Autodesk Inventor part; units mm, degrees
(part 6 of 6)
  line L4439 (-10.0121, 28.4168) -> (-10.0047, 28.6447)
  line L4440 (-10.0047, 28.6447) -> (-9.9918, 28.8863)
  line L4441 (-9.9918, 28.8863) -> (-9.973, 29.1388)
  line L4442 (-9.973, 29.1388) -> (-9.9523, 29.359)
  arc A136 (-9.2052, 29.6018) -> (-9.9523, 29.359) centre (0, 0) ccw
  line L4443 (-9.2052, 29.6018) -> (-9.059, 29.4358)
  line L4444 (-9.059, 29.4358) -> (-8.8954, 29.2425)
  line L4445 (-8.8954, 29.2425) -> (-8.7429, 29.0547)
  line L4446 (-8.7429, 29.0547) -> (-8.603, 28.8746)
  line L4447 (-8.603, 28.8746) -> (-8.4737, 28.7009)
  line L4448 (-8.4737, 28.7009) -> (-8.3547, 28.5338)
  line L4449 (-8.3547, 28.5338) -> (-8.2472, 28.3759)
  line L4450 (-8.2472, 28.3759) -> (-8.1494, 28.2257)
  line L4451 (-8.1494, 28.2257) -> (-7.9652, 27.9266)
  line L4452 (-7.9652, 27.9266) -> (-7.9351, 27.8907)
  line L4453 (-7.9351, 27.8907) -> (-7.9073, 27.8683)
  line L4454 (-7.9073, 27.8683) -> (-7.8823, 27.8592)
  line L4455 (-7.8823, 27.8592) -> (-7.8657, 27.861)
  line L4456 (-7.8657, 27.861) -> (-7.4928, 27.9636)
  line L4457 (-7.4928, 27.9636) -> (-7.1186, 28.0612)
  line L4458 (-7.1186, 28.0612) -> (-7.1033, 28.0679)
  line L4459 (-7.1033, 28.0679) -> (-7.0862, 28.0883)
  line L4460 (-7.0862, 28.0883) -> (-7.0733, 28.1216)
  line L4461 (-7.0733, 28.1216) -> (-7.0652, 28.1677)
  line L4462 (-7.0652, 28.1677) -> (-7.0553, 28.5189)
  line L4463 (-7.0553, 28.5189) -> (-7.0457, 28.6979)
  line L4464 (-7.0457, 28.6979) -> (-7.0315, 28.8883)
  line L4465 (-7.0315, 28.8883) -> (-7.012, 29.0926)
  line L4466 (-7.012, 29.0926) -> (-6.9869, 29.3077)
  line L4467 (-6.9869, 29.3077) -> (-6.9557, 29.5336)
  line L4468 (-6.9557, 29.5336) -> (-6.9177, 29.7725)
  line L4469 (-6.9177, 29.7725) -> (-6.8726, 30.0216)
  line L4470 (-6.8726, 30.0216) -> (-6.829, 30.2385)
  arc A137 (-6.0605, 30.4018) -> (-6.829, 30.2385) centre (0, 0) ccw
  line L4471 (-6.0605, 30.4018) -> (-5.9325, 30.2214)
  line L4472 (-5.9325, 30.2214) -> (-5.79, 30.0122)
  line L4473 (-5.79, 30.0122) -> (-5.658, 29.8094)
  line L4474 (-5.658, 29.8094) -> (-5.5376, 29.6157)
  line L4475 (-5.5376, 29.6157) -> (-5.4272, 29.4294)
  line L4476 (-5.4272, 29.4294) -> (-5.3263, 29.2508)
  line L4477 (-5.3263, 29.2508) -> (-5.2359, 29.0826)
  line L4478 (-5.2359, 29.0826) -> (-5.1544, 28.9229)
  line L4479 (-5.1544, 28.9229) -> (-5.0025, 28.6062)
  line L4480 (-5.0025, 28.6062) -> (-4.9763, 28.5674)
  line L4481 (-4.9763, 28.5674) -> (-4.951, 28.5421)
  line L4482 (-4.951, 28.5421) -> (-4.927, 28.5305)
  line L4483 (-4.927, 28.5305) -> (-4.9104, 28.5306)
  line L4484 (-4.9104, 28.5306) -> (-4.5288, 28.5936)
  line L4485 (-4.5288, 28.5936) -> (-4.1464, 28.6516)
  line L4486 (-4.1464, 28.6516) -> (-4.1305, 28.6567)
  line L4487 (-4.1305, 28.6567) -> (-4.1114, 28.6751)
  line L4488 (-4.1114, 28.6751) -> (-4.0951, 28.7069)
  line L4489 (-4.0951, 28.7069) -> (-4.0822, 28.7519)
  line L4490 (-4.0822, 28.7519) -> (-4.0356, 29.1001)
  line L4491 (-4.0356, 29.1001) -> (-4.0074, 29.2771)
  line L4492 (-4.0074, 29.2771) -> (-3.9734, 29.465)
  line L4493 (-3.9734, 29.465) -> (-3.9326, 29.6661)
  line L4494 (-3.9326, 29.6661) -> (-3.8852, 29.8774)
  line L4495 (-3.8852, 29.8774) -> (-3.8305, 30.0989)
  line L4496 (-3.8305, 30.0989) -> (-3.7677, 30.3325)
  line L4497 (-3.7677, 30.3325) -> (-3.6968, 30.5755)
  line L4498 (-3.6968, 30.5755) -> (-3.6308, 30.7866)
  arc A138 (-2.8495, 30.8688) -> (-3.6308, 30.7866) centre (0, 0) ccw
  line L4499 (-2.8495, 30.8688) -> (-2.741, 30.676)
  line L4500 (-2.741, 30.676) -> (-2.6211, 30.453)
  line L4501 (-2.6211, 30.453) -> (-2.5111, 30.2376)
  line L4502 (-2.5111, 30.2376) -> (-2.4116, 30.0323)
  line L4503 (-2.4116, 30.0323) -> (-2.3213, 29.8355)
  line L4504 (-2.3213, 29.8355) -> (-2.2396, 29.6473)
  line L4505 (-2.2396, 29.6473) -> (-2.1673, 29.4705)
  line L4506 (-2.1673, 29.4705) -> (-2.1029, 29.3033)
  line L4507 (-2.1029, 29.3033) -> (-1.9849, 28.9724)
  line L4508 (-1.9849, 28.9724) -> (-1.9629, 28.931)
  line L4509 (-1.9629, 28.931) -> (-1.9404, 28.9033)
  line L4510 (-1.9404, 28.9033) -> (-1.9178, 28.8892)
  line L4511 (-1.9178, 28.8892) -> (-1.9012, 28.8876)
  line L4512 (-1.9012, 28.8876) -> (-1.5151, 28.9103)
  line L4513 (-1.5151, 28.9103) -> (-1.1288, 28.9281)
  line L4514 (-1.1288, 28.9281) -> (-1.1124, 28.9314)
  line L4515 (-1.1124, 28.9314) -> (-1.0915, 28.9478)
  line L4516 (-1.0915, 28.9478) -> (-1.0719, 28.9777)
  line L4517 (-1.0719, 28.9777) -> (-1.0544, 29.0211)
  line L4518 (-1.0544, 29.0211) -> (-0.9717, 29.3626)
  line L4519 (-0.9717, 29.3626) -> (-0.9251, 29.5356)
  line L4520 (-0.9251, 29.5356) -> (-0.8717, 29.719)
  line L4521 (-0.8717, 29.719) -> (-0.8101, 29.9147)
  line L4522 (-0.8101, 29.9147) -> (-0.7408, 30.1199)
  line L4523 (-0.7408, 30.1199) -> (-0.6634, 30.3344)
  line L4524 (-0.6634, 30.3344) -> (-0.5765, 30.5601)
  line L4525 (-0.5765, 30.5601) -> (-0.4805, 30.7945)
  line L4526 (-0.4805, 30.7945) -> (-0.3928, 30.9975)
  arc A139 (0.3928, 30.9975) -> (-0.3928, 30.9975) centre (0, 0) ccw
  line L4527 (0.3928, 30.9975) -> (0.4805, 30.7945)
  line L4528 (0.4805, 30.7945) -> (0.5765, 30.5601)
  line L4529 (0.5765, 30.5601) -> (0.6634, 30.3344)
  line L4530 (0.6634, 30.3344) -> (0.7408, 30.1199)
  line L4531 (0.7408, 30.1199) -> (0.8101, 29.9147)
  line L4532 (0.8101, 29.9147) -> (0.8717, 29.719)
  line L4533 (0.8717, 29.719) -> (0.9251, 29.5356)
  line L4534 (0.9251, 29.5356) -> (0.9717, 29.3626)
  line L4535 (0.9717, 29.3626) -> (1.0544, 29.0211)
  line L4536 (1.0544, 29.0211) -> (1.0719, 28.9777)
  line L4537 (1.0719, 28.9777) -> (1.0915, 28.9478)
  line L4538 (1.0915, 28.9478) -> (1.1124, 28.9314)
  line L4539 (1.1124, 28.9314) -> (1.1288, 28.9281)
  line L4540 (1.1288, 28.9281) -> (1.5151, 28.9103)
  line L4541 (1.5151, 28.9103) -> (1.9012, 28.8876)
  line L4542 (1.9012, 28.8876) -> (1.9178, 28.8892)
  line L4543 (1.9178, 28.8892) -> (1.9404, 28.9033)
  line L4544 (1.9404, 28.9033) -> (1.9629, 28.931)
  line L4545 (1.9629, 28.931) -> (1.9849, 28.9724)
  line L4546 (1.9849, 28.9724) -> (2.1029, 29.3033)
  line L4547 (2.1029, 29.3033) -> (2.1673, 29.4705)
  line L4548 (2.1673, 29.4705) -> (2.2396, 29.6473)
  line L4549 (2.2396, 29.6473) -> (2.3213, 29.8355)
  line L4550 (2.3213, 29.8355) -> (2.4116, 30.0323)
  line L4551 (2.4116, 30.0323) -> (2.5111, 30.2376)
  line L4552 (2.5111, 30.2376) -> (2.6211, 30.453)
  line L4553 (2.6211, 30.453) -> (2.741, 30.676)
  line L4554 (2.741, 30.676) -> (2.8495, 30.8688)
  arc A140 (3.6308, 30.7866) -> (2.8495, 30.8688) centre (0, 0) ccw
  line L4555 (3.6308, 30.7866) -> (3.6968, 30.5755)
  line L4556 (3.6968, 30.5755) -> (3.7677, 30.3325)
  line L4557 (3.7677, 30.3325) -> (3.8305, 30.0989)
  line L4558 (3.8305, 30.0989) -> (3.8852, 29.8774)
  line L4559 (3.8852, 29.8774) -> (3.9326, 29.6661)
  line L4560 (3.9326, 29.6661) -> (3.9734, 29.465)
  line L4561 (3.9734, 29.465) -> (4.0074, 29.2771)
  line L4562 (4.0074, 29.2771) -> (4.0356, 29.1001)
  line L4563 (4.0356, 29.1001) -> (4.0822, 28.7519)
  line L4564 (4.0822, 28.7519) -> (4.0951, 28.7069)
  line L4565 (4.0951, 28.7069) -> (4.1114, 28.6751)
  line L4566 (4.1114, 28.6751) -> (4.1305, 28.6567)
  line L4567 (4.1305, 28.6567) -> (4.1464, 28.6516)
  line L4568 (4.1464, 28.6516) -> (4.5288, 28.5936)
  line L4569 (4.5288, 28.5936) -> (4.9104, 28.5306)
  line L4570 (4.9104, 28.5306) -> (4.927, 28.5305)
  line L4571 (4.927, 28.5305) -> (4.951, 28.5421)
  line L4572 (4.951, 28.5421) -> (4.9763, 28.5674)
  line L4573 (4.9763, 28.5674) -> (5.0025, 28.6062)
  line L4574 (5.0025, 28.6062) -> (5.1544, 28.9229)
  line L4575 (5.1544, 28.9229) -> (5.2359, 29.0826)
  line L4576 (5.2359, 29.0826) -> (5.3263, 29.2508)
  line L4577 (5.3263, 29.2508) -> (5.4272, 29.4294)
  line L4578 (5.4272, 29.4294) -> (5.5376, 29.6157)
  line L4579 (5.5376, 29.6157) -> (5.658, 29.8094)
  line L4580 (5.658, 29.8094) -> (5.79, 30.0122)
  line L4581 (5.79, 30.0122) -> (5.9325, 30.2214)
  line L4582 (5.9325, 30.2214) -> (6.0605, 30.4018)
  arc A141 (6.829, 30.2385) -> (6.0605, 30.4018) centre (0, 0) ccw
  line L4583 (6.829, 30.2385) -> (6.8726, 30.0216)
  line L4584 (6.8726, 30.0216) -> (6.9177, 29.7725)
  line L4585 (6.9177, 29.7725) -> (6.9557, 29.5336)
  line L4586 (6.9557, 29.5336) -> (6.9869, 29.3077)
  line L4587 (6.9869, 29.3077) -> (7.012, 29.0926)
  line L4588 (7.012, 29.0926) -> (7.0315, 28.8883)
  line L4589 (7.0315, 28.8883) -> (7.0457, 28.6979)
  line L4590 (7.0457, 28.6979) -> (7.0553, 28.5189)
  line L4591 (7.0553, 28.5189) -> (7.0652, 28.1677)
  line L4592 (7.0652, 28.1677) -> (7.0733, 28.1216)
  line L4593 (7.0733, 28.1216) -> (7.0862, 28.0883)
  line L4594 (7.0862, 28.0883) -> (7.1033, 28.0679)
  line L4595 (7.1033, 28.0679) -> (7.1186, 28.0612)
  line L4596 (7.1186, 28.0612) -> (7.4928, 27.9636)
  line L4597 (7.4928, 27.9636) -> (7.8657, 27.861)
  line L4598 (7.8657, 27.861) -> (7.8823, 27.8592)
  line L4599 (7.8823, 27.8592) -> (7.9073, 27.8683)
  line L4600 (7.9073, 27.8683) -> (7.9351, 27.8907)
  line L4601 (7.9351, 27.8907) -> (7.9652, 27.9266)
  line L4602 (7.9652, 27.9266) -> (8.1494, 28.2257)
  line L4603 (8.1494, 28.2257) -> (8.2472, 28.3759)
  line L4604 (8.2472, 28.3759) -> (8.3547, 28.5338)
  line L4605 (8.3547, 28.5338) -> (8.4737, 28.7009)
  line L4606 (8.4737, 28.7009) -> (8.603, 28.8746)
  line L4607 (8.603, 28.8746) -> (8.7429, 29.0547)
  line L4608 (8.7429, 29.0547) -> (8.8954, 29.2425)
  line L4609 (8.8954, 29.2425) -> (9.059, 29.4358)
  line L4610 (9.059, 29.4358) -> (9.2052, 29.6018)
  arc A142 (9.9523, 29.359) -> (9.2052, 29.6018) centre (0, 0) ccw
  line L4611 (9.9523, 29.359) -> (9.973, 29.1388)
  line L4612 (9.973, 29.1388) -> (9.9918, 28.8863)
  line L4613 (9.9918, 28.8863) -> (10.0047, 28.6447)
  line L4614 (10.0047, 28.6447) -> (10.0121, 28.4168)
  line L4615 (10.0121, 28.4168) -> (10.0146, 28.2002)
  line L4616 (10.0146, 28.2002) -> (10.0127, 27.995)
  line L4617 (10.0127, 27.995) -> (10.0069, 27.8042)
  line L4618 (10.0069, 27.8042) -> (9.9977, 27.6252)
  line L4619 (9.9977, 27.6252) -> (9.9708, 27.2749)
  line L4620 (9.9708, 27.2749) -> (9.9741, 27.2282)
  line L4621 (9.9741, 27.2282) -> (9.9834, 27.1937)
  line L4622 (9.9834, 27.1937) -> (9.9983, 27.1717)
  line L4623 (9.9983, 27.1717) -> (10.0128, 27.1634)
  line L4624 (10.0128, 27.1634) -> (10.3748, 27.0272)
  line L4625 (10.3748, 27.0272) -> (10.7349, 26.8862)
  line L4626 (10.7349, 26.8862) -> (10.7512, 26.8826)
  line L4627 (10.7512, 26.8826) -> (10.777, 26.8891)
  line L4628 (10.777, 26.8891) -> (10.807, 26.9085)
  line L4629 (10.807, 26.9085) -> (10.8407, 26.941)
  line L4630 (10.8407, 26.941) -> (11.0551, 27.2193)
  line L4631 (11.0551, 27.2193) -> (11.1681, 27.3584)
  line L4632 (11.1681, 27.3584) -> (11.2915, 27.5042)
  line L4633 (11.2915, 27.5042) -> (11.4273, 27.6579)
  line L4634 (11.4273, 27.6579) -> (11.5741, 27.8172)
  line L4635 (11.5741, 27.8172) -> (11.7321, 27.9817)
  line L4636 (11.7321, 27.9817) -> (11.9033, 28.1525)
  line L4637 (11.9033, 28.1525) -> (12.0862, 28.3276)
  line L4638 (12.0862, 28.3276) -> (12.249, 28.4774)
  arc A143 (12.9667, 28.1579) -> (12.249, 28.4774) centre (0, 0) ccw
  line L4639 (12.9667, 28.1579) -> (12.9642, 27.9367)
  line L4640 (12.9642, 27.9367) -> (12.9565, 27.6836)
  line L4641 (12.9565, 27.6836) -> (12.9441, 27.442)
  line L4642 (12.9441, 27.442) -> (12.9276, 27.2145)
  line L4643 (12.9276, 27.2145) -> (12.9075, 26.9989)
  line L4644 (12.9075, 26.9989) -> (12.8841, 26.7951)
  line L4645 (12.8841, 26.7951) -> (12.8584, 26.6059)
  line L4646 (12.8584, 26.6059) -> (12.8305, 26.4288)
  line L4647 (12.8305, 26.4288) -> (12.7672, 26.0833)
  line L4648 (12.7672, 26.0833) -> (12.7656, 26.0365)
  line L4649 (12.7656, 26.0365) -> (12.7712, 26.0012)
  line L4650 (12.7712, 26.0012) -> (12.7837, 25.9777)
  line L4651 (12.7837, 25.9777) -> (12.7973, 25.968)
  line L4652 (12.7973, 25.968) -> (13.143, 25.7946)
  line L4653 (13.143, 25.7946) -> (13.4865, 25.6168)
  line L4654 (13.4865, 25.6168) -> (13.5023, 25.6116)
  line L4655 (13.5023, 25.6116) -> (13.5287, 25.6153)
  line L4656 (13.5287, 25.6153) -> (13.5605, 25.6314)
  line L4657 (13.5605, 25.6314) -> (13.5974, 25.6603)
  line L4658 (13.5974, 25.6603) -> (13.8398, 25.9146)
  line L4659 (13.8398, 25.9146) -> (13.9666, 26.0412)
  line L4660 (13.9666, 26.0412) -> (14.1046, 26.1732)
  line L4661 (14.1046, 26.1732) -> (14.2558, 26.312)
  line L4662 (14.2558, 26.312) -> (14.4184, 26.455)
  line L4663 (14.4184, 26.455) -> (14.5927, 26.602)
  line L4664 (14.5927, 26.602) -> (14.7808, 26.7541)
  line L4665 (14.7808, 26.7541) -> (14.9811, 26.9091)
  line L4666 (14.9811, 26.9091) -> (15.1586, 27.041)
  arc A144 (15.8389, 26.6482) -> (15.1586, 27.041) centre (0, 0) ccw
  line L4667 (15.8389, 26.6482) -> (15.8134, 26.4285)
  line L4668 (15.8134, 26.4285) -> (15.7793, 26.1776)
  line L4669 (15.7793, 26.1776) -> (15.7417, 25.9387)
  line L4670 (15.7417, 25.9387) -> (15.7015, 25.7142)
  line L4671 (15.7015, 25.7142) -> (15.6589, 25.5018)
  line L4672 (15.6589, 25.5018) -> (15.6144, 25.3015)
  line L4673 (15.6144, 25.3015) -> (15.569, 25.1161)
  line L4674 (15.569, 25.1161) -> (15.5228, 24.9429)
  line L4675 (15.5228, 24.9429) -> (15.4237, 24.6058)
  line L4676 (15.4237, 24.6058) -> (15.4172, 24.5595)
  line L4677 (15.4172, 24.5595) -> (15.4191, 24.5238)
  line L4678 (15.4191, 24.5238) -> (15.4291, 24.4991)
  line L4679 (15.4291, 24.4991) -> (15.4416, 24.488)
  line L4680 (15.4416, 24.488) -> (15.7673, 24.2795)
  line L4681 (15.7673, 24.2795) -> (16.0903, 24.0668)
  line L4682 (16.0903, 24.0668) -> (16.1055, 24.0599)
  line L4683 (16.1055, 24.0599) -> (16.1321, 24.0608)
  line L4684 (16.1321, 24.0608) -> (16.1655, 24.0735)
  line L4685 (16.1655, 24.0735) -> (16.2052, 24.0984)
  line L4686 (16.2052, 24.0984) -> (16.4728, 24.326)
  line L4687 (16.4728, 24.326) -> (16.6122, 24.4386)
  line L4688 (16.6122, 24.4386) -> (16.7632, 24.5555)
  line L4689 (16.7632, 24.5555) -> (16.928, 24.6777)
  line L4690 (16.928, 24.6777) -> (17.1047, 24.8029)
  line L4691 (17.1047, 24.8029) -> (17.2934, 24.931)
  line L4692 (17.2934, 24.931) -> (17.4964, 25.0625)
  line L4693 (17.4964, 25.0625) -> (17.7118, 25.1957)
  line L4694 (17.7118, 25.1957) -> (17.9021, 25.3084)
  arc A145 (18.5377, 24.8466) -> (17.9021, 25.3084) centre (0, 0) ccw
  line L4695 (18.5377, 24.8466) -> (18.4893, 24.6308)
  line L4696 (18.4893, 24.6308) -> (18.4292, 24.3848)
  line L4697 (18.4292, 24.3848) -> (18.3668, 24.1511)
  line L4698 (18.3668, 24.1511) -> (18.3034, 23.932)
  line L4699 (18.3034, 23.932) -> (18.2388, 23.7253)
  line L4700 (18.2388, 23.7253) -> (18.1736, 23.5308)
  line L4701 (18.1736, 23.5308) -> (18.1091, 23.3511)
  line L4702 (18.1091, 23.3511) -> (18.045, 23.1837)
  line L4703 (18.045, 23.1837) -> (17.9112, 22.8588)
  line L4704 (17.9112, 22.8588) -> (17.8999, 22.8134)
  line L4705 (17.8999, 22.8134) -> (17.8981, 22.7777)
  line L4706 (17.8981, 22.7777) -> (17.9055, 22.7521)
  line L4707 (17.9055, 22.7521) -> (17.9167, 22.7398)
  line L4708 (17.9167, 22.7398) -> (18.2188, 22.4984)
  line L4709 (18.2188, 22.4984) -> (18.5178, 22.2531)
  line L4710 (18.5178, 22.2531) -> (18.5322, 22.2446)
  line L4711 (18.5322, 22.2446) -> (18.5587, 22.2427)
  line L4712 (18.5587, 22.2427) -> (18.5933, 22.2519)
  line L4713 (18.5933, 22.2519) -> (18.6353, 22.2724)
  line L4714 (18.6353, 22.2724) -> (18.9253, 22.4708)
  line L4715 (18.9253, 22.4708) -> (19.0757, 22.5683)
  line L4716 (19.0757, 22.5683) -> (19.2381, 22.6688)
  line L4717 (19.2381, 22.6688) -> (19.4148, 22.773)
  line L4718 (19.4148, 22.773) -> (19.6036, 22.8791)
  line L4719 (19.6036, 22.8791) -> (19.8047, 22.9867)
  line L4720 (19.8047, 22.9867) -> (20.0203, 23.0963)
  line L4721 (20.0203, 23.0963) -> (20.2484, 23.2063)
  line L4722 (20.2484, 23.2063) -> (20.4495, 23.2985)
  arc A146 (21.0333, 22.7728) -> (20.4495, 23.2985) centre (0, 0) ccw
  line L4723 (21.0333, 22.7728) -> (20.9626, 22.5632)
  line L4724 (20.9626, 22.5632) -> (20.8771, 22.3249)
  line L4725 (20.8771, 22.3249) -> (20.7906, 22.099)
  line L4726 (20.7906, 22.099) -> (20.7047, 21.8877)
  line L4727 (20.7047, 21.8877) -> (20.6189, 21.6889)
  line L4728 (20.6189, 21.6889) -> (20.5336, 21.5022)
  line L4729 (20.5336, 21.5022) -> (20.4507, 21.3302)
  line L4730 (20.4507, 21.3302) -> (20.3695, 21.1705)
  line L4731 (20.3695, 21.1705) -> (20.2025, 20.8614)
  line L4732 (20.2025, 20.8614) -> (20.1865, 20.8174)
  line L4733 (20.1865, 20.8174) -> (20.181, 20.7821)
  line L4734 (20.181, 20.7821) -> (20.1856, 20.7559)
  line L4735 (20.1856, 20.7559) -> (20.1955, 20.7424)
  line L4736 (20.1955, 20.7424) -> (20.4707, 20.4707)
  line L4737 (20.4707, 20.4707) -> (20.7424, 20.1955)
  line L4738 (20.7424, 20.1955) -> (20.7559, 20.1856)
  line L4739 (20.7559, 20.1856) -> (20.7821, 20.181)
  line L4740 (20.7821, 20.181) -> (20.8174, 20.1865)
  line L4741 (20.8174, 20.1865) -> (20.8614, 20.2025)
  line L4742 (20.8614, 20.2025) -> (21.1705, 20.3695)
  line L4743 (21.1705, 20.3695) -> (21.3302, 20.4507)
  line L4744 (21.3302, 20.4507) -> (21.5022, 20.5336)
  line L4745 (21.5022, 20.5336) -> (21.6889, 20.6189)
  line L4746 (21.6889, 20.6189) -> (21.8877, 20.7047)
  line L4747 (21.8877, 20.7047) -> (22.099, 20.7906)
  line L4748 (22.099, 20.7906) -> (22.3249, 20.8771)
  line L4749 (22.3249, 20.8771) -> (22.5632, 20.9626)
  line L4750 (22.5632, 20.9626) -> (22.7728, 21.0333)
  arc A147 (23.2985, 20.4495) -> (22.7728, 21.0333) centre (0, 0) ccw
  line L4751 (23.2985, 20.4495) -> (23.2063, 20.2484)
  line L4752 (23.2063, 20.2484) -> (23.0963, 20.0203)
  line L4753 (23.0963, 20.0203) -> (22.9867, 19.8047)
  line L4754 (22.9867, 19.8047) -> (22.8791, 19.6036)
  line L4755 (22.8791, 19.6036) -> (22.773, 19.4148)
  line L4756 (22.773, 19.4148) -> (22.6688, 19.2381)
  line L4757 (22.6688, 19.2381) -> (22.5683, 19.0757)
  line L4758 (22.5683, 19.0757) -> (22.4708, 18.9253)
  line L4759 (22.4708, 18.9253) -> (22.2724, 18.6353)
  line L4760 (22.2724, 18.6353) -> (22.2519, 18.5933)
  line L4761 (22.2519, 18.5933) -> (22.2427, 18.5587)
  line L4762 (22.2427, 18.5587) -> (22.2446, 18.5322)
  line L4763 (22.2446, 18.5322) -> (22.2531, 18.5178)
  line L4764 (22.2531, 18.5178) -> (22.4984, 18.2188)
  line L4765 (22.4984, 18.2188) -> (22.7398, 17.9167)
  line L4766 (22.7398, 17.9167) -> (22.7521, 17.9055)
  line L4767 (22.7521, 17.9055) -> (22.7777, 17.8981)
  line L4768 (22.7777, 17.8981) -> (22.8134, 17.8999)
  line L4769 (22.8134, 17.8999) -> (22.8588, 17.9112)
  line L4770 (22.8588, 17.9112) -> (23.1837, 18.045)
  line L4771 (23.1837, 18.045) -> (23.3511, 18.1091)
  line L4772 (23.3511, 18.1091) -> (23.5308, 18.1736)
  line L4773 (23.5308, 18.1736) -> (23.7253, 18.2388)
  line L4774 (23.7253, 18.2388) -> (23.932, 18.3034)
  line L4775 (23.932, 18.3034) -> (24.1511, 18.3668)
  line L4776 (24.1511, 18.3668) -> (24.3848, 18.4292)
  line L4777 (24.3848, 18.4292) -> (24.6308, 18.4893)
  line L4778 (24.6308, 18.4893) -> (24.8466, 18.5377)
  arc A148 (25.3084, 17.9021) -> (24.8466, 18.5377) centre (0, 0) ccw
  line L4779 (25.3084, 17.9021) -> (25.1957, 17.7118)
  line L4780 (25.1957, 17.7118) -> (25.0625, 17.4964)
  line L4781 (25.0625, 17.4964) -> (24.931, 17.2934)
  line L4782 (24.931, 17.2934) -> (24.8029, 17.1047)
  line L4783 (24.8029, 17.1047) -> (24.6777, 16.928)
  line L4784 (24.6777, 16.928) -> (24.5555, 16.7632)
  line L4785 (24.5555, 16.7632) -> (24.4386, 16.6122)
  line L4786 (24.4386, 16.6122) -> (24.326, 16.4728)
  line L4787 (24.326, 16.4728) -> (24.0984, 16.2052)
  line L4788 (24.0984, 16.2052) -> (24.0735, 16.1655)
  line L4789 (24.0735, 16.1655) -> (24.0608, 16.1321)
  line L4790 (24.0608, 16.1321) -> (24.0599, 16.1055)
  line L4791 (24.0599, 16.1055) -> (24.0668, 16.0903)
  line L4792 (24.0668, 16.0903) -> (24.2795, 15.7673)
  line L4793 (24.2795, 15.7673) -> (24.488, 15.4416)
  line L4794 (24.488, 15.4416) -> (24.4991, 15.4291)
  line L4795 (24.4991, 15.4291) -> (24.5238, 15.4191)
  line L4796 (24.5238, 15.4191) -> (24.5595, 15.4172)
  line L4797 (24.5595, 15.4172) -> (24.6058, 15.4237)
  line L4798 (24.6058, 15.4237) -> (24.9429, 15.5228)
  line L4799 (24.9429, 15.5228) -> (25.1161, 15.569)
  line L4800 (25.1161, 15.569) -> (25.3015, 15.6144)
  line L4801 (25.3015, 15.6144) -> (25.5018, 15.6589)
  line L4802 (25.5018, 15.6589) -> (25.7142, 15.7015)
  line L4803 (25.7142, 15.7015) -> (25.9387, 15.7417)
  line L4804 (25.9387, 15.7417) -> (26.1776, 15.7793)
  line L4805 (26.1776, 15.7793) -> (26.4285, 15.8134)
  line L4806 (26.4285, 15.8134) -> (26.6482, 15.8389)
  arc A149 (27.041, 15.1586) -> (26.6482, 15.8389) centre (0, 0) ccw
  line L4807 (27.041, 15.1586) -> (26.9091, 14.9811)
  line L4808 (26.9091, 14.9811) -> (26.7541, 14.7808)
  line L4809 (26.7541, 14.7808) -> (26.602, 14.5927)
  line L4810 (26.602, 14.5927) -> (26.455, 14.4184)
  line L4811 (26.455, 14.4184) -> (26.312, 14.2558)
  line L4812 (26.312, 14.2558) -> (26.1732, 14.1046)
  line L4813 (26.1732, 14.1046) -> (26.0412, 13.9666)
  line L4814 (26.0412, 13.9666) -> (25.9146, 13.8398)
  line L4815 (25.9146, 13.8398) -> (25.6603, 13.5974)
  line L4816 (25.6603, 13.5974) -> (25.6314, 13.5605)
  line L4817 (25.6314, 13.5605) -> (25.6153, 13.5287)
  line L4818 (25.6153, 13.5287) -> (25.6116, 13.5023)
  line L4819 (25.6116, 13.5023) -> (25.6168, 13.4865)
  line L4820 (25.6168, 13.4865) -> (25.7946, 13.143)
  line L4821 (25.7946, 13.143) -> (25.968, 12.7973)
  line L4822 (25.968, 12.7973) -> (25.9777, 12.7837)
  line L4823 (25.9777, 12.7837) -> (26.0012, 12.7712)
  line L4824 (26.0012, 12.7712) -> (26.0365, 12.7656)
  line L4825 (26.0365, 12.7656) -> (26.0833, 12.7672)
  line L4826 (26.0833, 12.7672) -> (26.4288, 12.8305)
  line L4827 (26.4288, 12.8305) -> (26.6059, 12.8584)
  line L4828 (26.6059, 12.8584) -> (26.7951, 12.8841)
  line L4829 (26.7951, 12.8841) -> (26.9989, 12.9075)
  line L4830 (26.9989, 12.9075) -> (27.2145, 12.9276)
  line L4831 (27.2145, 12.9276) -> (27.442, 12.9441)
  line L4832 (27.442, 12.9441) -> (27.6836, 12.9565)
  line L4833 (27.6836, 12.9565) -> (27.9367, 12.9642)
  line L4834 (27.9367, 12.9642) -> (28.1579, 12.9667)
  arc A150 (28.4774, 12.249) -> (28.1579, 12.9667) centre (0, 0) ccw
  line L4835 (28.4774, 12.249) -> (28.3276, 12.0862)
  line L4836 (28.3276, 12.0862) -> (28.1525, 11.9033)
  line L4837 (28.1525, 11.9033) -> (27.9817, 11.7321)
  line L4838 (27.9817, 11.7321) -> (27.8172, 11.5741)
  line L4839 (27.8172, 11.5741) -> (27.6579, 11.4273)
  line L4840 (27.6579, 11.4273) -> (27.5042, 11.2915)
  line L4841 (27.5042, 11.2915) -> (27.3584, 11.1681)
  line L4842 (27.3584, 11.1681) -> (27.2193, 11.0551)
  line L4843 (27.2193, 11.0551) -> (26.941, 10.8407)
  line L4844 (26.941, 10.8407) -> (26.9085, 10.807)
  line L4845 (26.9085, 10.807) -> (26.8891, 10.777)
  line L4846 (26.8891, 10.777) -> (26.8826, 10.7512)
  line L4847 (26.8826, 10.7512) -> (26.8862, 10.7349)
  line L4848 (26.8862, 10.7349) -> (27.0272, 10.3748)
  line L4849 (27.0272, 10.3748) -> (27.1634, 10.0128)
  line L4850 (27.1634, 10.0128) -> (27.1717, 9.9983)
  line L4851 (27.1717, 9.9983) -> (27.1937, 9.9834)
  line L4852 (27.1937, 9.9834) -> (27.2282, 9.9741)
  line L4853 (27.2282, 9.9741) -> (27.2749, 9.9708)
  line L4854 (27.2749, 9.9708) -> (27.6252, 9.9977)
  line L4855 (27.6252, 9.9977) -> (27.8042, 10.0069)
  line L4856 (27.8042, 10.0069) -> (27.995, 10.0127)
  line L4857 (27.995, 10.0127) -> (28.2002, 10.0146)
  line L4858 (28.2002, 10.0146) -> (28.4168, 10.0121)
  line L4859 (28.4168, 10.0121) -> (28.6447, 10.0047)
  line L4860 (28.6447, 10.0047) -> (28.8863, 9.9918)
  line L4861 (28.8863, 9.9918) -> (29.1388, 9.973)
  line L4862 (29.1388, 9.973) -> (29.359, 9.9523)
  arc A151 (29.6018, 9.2052) -> (29.359, 9.9523) centre (0, 0) ccw
  line L4863 (29.6018, 9.2052) -> (29.4358, 9.059)
  line L4864 (29.4358, 9.059) -> (29.2425, 8.8954)
  line L4865 (29.2425, 8.8954) -> (29.0547, 8.7429)
  line L4866 (29.0547, 8.7429) -> (28.8746, 8.603)
  line L4867 (28.8746, 8.603) -> (28.7009, 8.4737)
  line L4868 (28.7009, 8.4737) -> (28.5338, 8.3547)
  line L4869 (28.5338, 8.3547) -> (28.3759, 8.2472)
  line L4870 (28.3759, 8.2472) -> (28.2257, 8.1494)
  line L4871 (28.2257, 8.1494) -> (27.9266, 7.9652)
  line L4872 (27.9266, 7.9652) -> (27.8907, 7.9351)
  line L4873 (27.8907, 7.9351) -> (27.8683, 7.9073)
  line L4874 (27.8683, 7.9073) -> (27.8592, 7.8823)
  line L4875 (27.8592, 7.8823) -> (27.861, 7.8657)
  line L4876 (27.861, 7.8657) -> (27.9636, 7.4928)
  line L4877 (27.9636, 7.4928) -> (28.0612, 7.1186)
  line L4878 (28.0612, 7.1186) -> (28.0679, 7.1033)
  line L4879 (28.0679, 7.1033) -> (28.0883, 7.0862)
  line L4880 (28.0883, 7.0862) -> (28.1216, 7.0733)
  line L4881 (28.1216, 7.0733) -> (28.1677, 7.0652)
  line L4882 (28.1677, 7.0652) -> (28.5189, 7.0553)
  line L4883 (28.5189, 7.0553) -> (28.6979, 7.0457)
  line L4884 (28.6979, 7.0457) -> (28.8883, 7.0315)
  line L4885 (28.8883, 7.0315) -> (29.0926, 7.012)
  line L4886 (29.0926, 7.012) -> (29.3077, 6.9869)
  line L4887 (29.3077, 6.9869) -> (29.5336, 6.9557)
  line L4888 (29.5336, 6.9557) -> (29.7725, 6.9177)
  line L4889 (29.7725, 6.9177) -> (30.0216, 6.8726)
  line L4890 (30.0216, 6.8726) -> (30.2385, 6.829)
  arc A152 (30.4018, 6.0605) -> (30.2385, 6.829) centre (0, 0) ccw
  line L4891 (30.4018, 6.0605) -> (30.2214, 5.9325)
  line L4892 (30.2214, 5.9325) -> (30.0122, 5.79)
  line L4893 (30.0122, 5.79) -> (29.8094, 5.658)
  line L4894 (29.8094, 5.658) -> (29.6157, 5.5376)
  line L4895 (29.6157, 5.5376) -> (29.4294, 5.4272)
  line L4896 (29.4294, 5.4272) -> (29.2508, 5.3263)
  line L4897 (29.2508, 5.3263) -> (29.0826, 5.2359)
  line L4898 (29.0826, 5.2359) -> (28.9229, 5.1544)
  line L4899 (28.9229, 5.1544) -> (28.6062, 5.0025)
  line L4900 (28.6062, 5.0025) -> (28.5674, 4.9763)
  line L4901 (28.5674, 4.9763) -> (28.5421, 4.951)
  line L4902 (28.5421, 4.951) -> (28.5305, 4.927)
  line L4903 (28.5305, 4.927) -> (28.5306, 4.9104)
  line L4904 (28.5306, 4.9104) -> (28.5936, 4.5288)
  line L4905 (28.5936, 4.5288) -> (28.6516, 4.1464)
  line L4906 (28.6516, 4.1464) -> (28.6567, 4.1305)
  line L4907 (28.6567, 4.1305) -> (28.6751, 4.1114)
  line L4908 (28.6751, 4.1114) -> (28.7069, 4.0951)
  line L4909 (28.7069, 4.0951) -> (28.7519, 4.0822)
  line L4910 (28.7519, 4.0822) -> (29.1001, 4.0356)
  line L4911 (29.1001, 4.0356) -> (29.2771, 4.0074)
  line L4912 (29.2771, 4.0074) -> (29.465, 3.9734)
  line L4913 (29.465, 3.9734) -> (29.6661, 3.9326)
  line L4914 (29.6661, 3.9326) -> (29.8774, 3.8852)
  line L4915 (29.8774, 3.8852) -> (30.0989, 3.8305)
  line L4916 (30.0989, 3.8305) -> (30.3325, 3.7677)
  line L4917 (30.3325, 3.7677) -> (30.5755, 3.6968)
  line L4918 (30.5755, 3.6968) -> (30.7866, 3.6308)
  arc A153 (30.8688, 2.8495) -> (30.7866, 3.6308) centre (0, 0) ccw
  line L4919 (30.8688, 2.8495) -> (30.676, 2.741)
  point P0 (30.8688, 2.8495)
  point P1 (30.7866, 3.6308)
  point P2 (30.4018, 6.0605)
  point P3 (30.2385, 6.829)
  point P4 (29.6018, 9.2052)
  point P5 (29.359, 9.9523)
  point P6 (28.4774, 12.249)
  point P7 (28.1579, 12.9667)
  point P8 (27.041, 15.1586)
  point P9 (26.6482, 15.8389)
  point P10 (25.3084, 17.9021)
  point P11 (24.8466, 18.5377)
  point P12 (23.2985, 20.4495)
  point P13 (22.7728, 21.0333)
  point P14 (21.0333, 22.7728)
  point P15 (20.4495, 23.2985)
  point P16 (18.5377, 24.8466)
  point P17 (17.9021, 25.3084)
  point P18 (15.8389, 26.6482)
  point P19 (15.1586, 27.041)
  point P20 (12.9667, 28.1579)
  point P21 (12.249, 28.4774)
  point P22 (9.9523, 29.359)
  point P23 (9.2052, 29.6018)
  point P24 (6.0605, 30.4018)
  point P25 (3.6308, 30.7866)
  point P26 (2.8495, 30.8688)
  point P27 (0.3928, 30.9975)
  point P28 (-0.3928, 30.9975)
  point P29 (-2.8495, 30.8688)
  point P30 (-3.6308, 30.7866)
  point P31 (-6.0605, 30.4018)
  point P32 (-6.829, 30.2385)
  point P33 (-9.2052, 29.6018)
  point P34 (-9.9523, 29.359)
  point P35 (-12.249, 28.4774)
  point P36 (-12.9667, 28.1579)
  point P37 (-15.1586, 27.041)
  point P38 (-15.8389, 26.6482)
  point P39 (-17.9021, 25.3084)
  point P40 (-18.5377, 24.8466)
  point P41 (-20.4495, 23.2985)
  point P42 (-21.0333, 22.7728)
  point P43 (-22.7728, 21.0333)
  point P44 (-23.2985, 20.4495)
  point P45 (-24.8466, 18.5377)
  point P46 (-25.3084, 17.9021)
  point P47 (-26.6482, 15.8389)
  point P48 (-27.041, 15.1586)
  point P49 (-28.1579, 12.9667)
  point P50 (-28.4774, 12.249)
  point P51 (-29.359, 9.9523)
  point P52 (-29.6018, 9.2052)
  point P53 (-30.4018, 6.0605)
  point P54 (-30.7866, 3.6308)
  point P55 (-30.8688, 2.8495)
  point P56 (-30.9975, 0.3928)
  point P57 (-30.9975, -0.3928)
  point P58 (-30.8688, -2.8495)
  point P59 (-30.7866, -3.6308)
  point P60 (-30.4018, -6.0605)
  point P61 (-30.2385, -6.829)
  point P62 (-29.6018, -9.2052)
  point P63 (-29.359, -9.9523)
  point P64 (-28.4774, -12.249)
  point P65 (-28.1579, -12.9667)
  point P66 (-27.041, -15.1586)
  point P67 (-26.6482, -15.8389)
  point P68 (-25.3084, -17.9021)
  point P69 (-24.8466, -18.5377)
  point P70 (-23.2985, -20.4495)
  point P71 (-22.7728, -21.0333)
  point P72 (-21.0333, -22.7728)
  point P73 (-20.4495, -23.2985)
  point P74 (-18.5377, -24.8466)
  point P75 (-17.9021, -25.3084)
  point P76 (-15.8389, -26.6482)
  point P77 (-15.1586, -27.041)
  point P78 (-12.9667, -28.1579)
  point P79 (-12.249, -28.4774)
  point P80 (-9.9523, -29.359)
  point P81 (-9.2052, -29.6018)
  point P82 (-6.829, -30.2385)
  point P83 (-6.0605, -30.4018)
  point P84 (-3.6308, -30.7866)
  point P85 (-2.8495, -30.8688)
  point P86 (-0.3928, -30.9975)
  point P87 (0.3928, -30.9975)
  point P88 (2.8495, -30.8688)
  point P89 (3.6308, -30.7866)
  point P90 (6.0605, -30.4018)
  point P91 (6.829, -30.2385)
  point P92 (9.2052, -29.6018)
  point P93 (9.9523, -29.359)
  point P94 (12.249, -28.4774)
  point P95 (12.9667, -28.1579)
  point P96 (15.1586, -27.041)
  point P97 (15.8389, -26.6482)
  point P98 (17.9021, -25.3084)
  point P99 (18.5377, -24.8466)
  point P100 (20.4495, -23.2985)
  point P101 (21.0333, -22.7728)
  point P102 (22.7728, -21.0333)
  point P103 (23.2985, -20.4495)
  point P104 (24.8466, -18.5377)
  point P105 (25.3084, -17.9021)
  point P106 (26.6482, -15.8389)
  point P107 (27.041, -15.1586)
  point P108 (28.1579, -12.9667)
  point P109 (28.4774, -12.249)
  point P110 (29.359, -9.9523)
  point P111 (29.6018, -9.2052)
  point P112 (30.2385, -6.829)
  point P113 (30.4018, -6.0605)
  point P114 (30.7866, -3.6308)
  point P115 (30.8688, -2.8495)
  point P116 (30.9975, -0.3928)
  point P117 (30.9975, 0.3928)
  point P118 (30.4357, -4.7271)
  point P119 (30.8213, -5.2578)
  point P120 (32.9691, -7.1917)
  point P121 (33.5372, -7.5197)
  point P122 (36.286, -8.4128)
  point P123 (36.9384, -8.4814)
  point P124 (39.8127, -8.1793)
  point P125 (40.4366, -7.9766)
  point P126 (42.9396, -6.5315)
  point P127 (43.4271, -6.0925)
  point P128 (45.1259, -3.7543)
  point P129 (45.3927, -3.155)
  point P130 (45.9936, -0.328)
  point P131 (45.9936, 0.328)
  point P132 (45.3927, 3.155)
  point P133 (45.1259, 3.7543)
  point P134 (43.4271, 6.0925)
  point P135 (42.9396, 6.5315)
  point P136 (40.4366, 7.9766)
  point P137 (39.8127, 8.1793)
  point P138 (36.9384, 8.4814)
  point P139 (36.286, 8.4128)
  point P140 (33.5372, 7.5197)
  point P141 (32.9691, 7.1917)
  point P142 (30.8213, 5.2578)
  point P143 (30.4357, 4.7271)
  point P144 (29.2602, 2.0868)
  point P145 (29.1238, 1.4451)
  point P146 (29.1238, -1.4451)
  point P147 (29.2602, -2.0868)
  constraints: 9840 end point, 300 point on circle, 154 centre point
extrude "Extrusion2" add sketch "Sketch1" along normal blind 5.55 contours L0 L1 L2 L3 L4 L5 L6 L7 L8 L9 L10 L11 L12 L13 L14 L15 L16 L17 L18 L19 L20 L21 L22 L23 L24 L25 L26 L27 L28 L29 L30 L31 L32 L33 L34 L35 L36 L37 L38 L39 L40 L41 L42 L43 L44 L45 L46 L47 L48 L49 L50 A4 L51 L52 L53 L54 L55 L56 L57 L58 L59 L60 L61 L62 L63 L64 L65 L66 L67 L68 L69 L70 L71 L72 L73 L74 L75 L76 L77 L78 L79 L80 L81 L82 L83 L84 L85 L86 L87 L88 L89 L90 L91 L92 L93 L94 L95 L96 L97 L98 L99 L100 L101 L102 A5 L103 L104 L105 L106 L107 L108 L109 L110 L111 L112 L113 L114 L115 L116 L117 L118 L119 L120 L121 L122 L123 L124 L125 L126 L127 L128 L129 L130 L131 L132 L133 L134 L135 L136 L137 L138 L139 L140 L141 L142 L143 L144 L145 L146 L147 L148 L149 L150 L151 L152 L153 L154 A6 L155 L156 L157 L158 L159 L160 L161 L162 L163 L164 L165 L166 L167 L168 L169 L170 L171 L172 L173 L174 L175 L176 L177 L178 L179 L180 L181 L182 L183 L184 L185 L186 L187 L188 L189 L190 L191 L192 L193 L194 L195 L196 L197 L198 L199 L200 L201 L202 L203 L204 L205 L206 A7 L207 L208 L209 L210 L211 L212 L213 L214 L215 L216 L217 L218 L219 L220 L221 L222 L223 L224 L225 L226 L227 L228 L229 L230 L231 L232 L233 L234 L235 L236 L237 L238 L239 L240 L241 L242 L243 L244 L245 L246 L247 L248 L249 L250 L251 L252 L253 L254 L255 L256 L257 L258 A8 L259 L260 L261 L262 L263 L264 L265 L266 L267 L268 L269 L270 L271 L272 L273 L274 L275 L276 L277 L278 L279 L280 L281 L282 L283 L284 L285 L286 L287 L288 L289 L290 L291 L292 L293 L294 L295 L296 L297 L298 L299 L300 L301 L302 L303 L304 L305 L306 L307 L308 L309 L310 A9 L311 L312 L313 L314 L315 L316 L317 L318 L319 L320 L321 L322 L323 L324 L325 L326 L327 L328 L329 L330 L331 L332 L333 L334 L335 L336 L337 L338 L339 L340 L341 L342 L343 L344 L345 L346 L347 L348 L349 L350 L351 L352 L353 L354 L355 L356 L357 L358 L359 L360 L361 L362 A10 L363 L364 L365 L366 L367 L368 L369 L370 L371 L372 L373 L374 L375 L376 L377 L378 L379 L380 L381 L382 L383 L384 L385 L386 L387 L388 L389 L390 L391 L392 L393 L394 L395 L396 L397 L398 L399 L400 L401 L402 L403 L404 L405 L406 L407 L408 L409 L410 L411 L412 L413 L414 A11 L415 L416 L417 L418 L419 L420 L421 L422 L423 L424 L425 L426 L427 L428 L429 L430 L431 L432 L433 L434 L435 L436 L437 L438 L439 L440 L441 L442 L443 L444 L445 L446 L447 L448 L449 L450 L451 L452 L453 L454 L455 L456 L457 L458 L459 L460 L461 L462 L463 L464 L465 L466 A12 L467 L468 L469 L470 L471 L472 L473 L474 L475 L476 L477 L478 L479 L480 L481 L482 L483 L484 L485 L486 L487 L488 L489 L490 L491 L492 L493 L494 L495 L496 L497 L498 L499 L500 L501 L502 L503 L504 L505 L506 L507 L508 L509 L510 L511 L512 L513 L514 L515 L516 L517 L518 A13 L519 L520 L521 L522 L523 L524 L525 L526 L527 L528 L529 L530 L531 L532 L533 L534 L535 L536 L537 L538 L539 L540 L541 L542 L543 L544 L545 L546 L547 L548 L549 L550 L551 L552 L553 L554 L555 L556 L557 L558 L559 L560 L561 L562 L563 L564 L565 L566 L567 L568 L569 L570 A14 L571 L572 L573 L574 L575 L576 L577 L578 L579 L580 L581 L582 L583 L584 L585 L586 L587 L588 L589 L590 L591 L592 L593 L594 L595 L596 L597 L598 L599 L600 L601 L602 L603 L604 L605 L606 L607 L608 L609 L610 L611 L612 L613 L614 L615 L616 L617 L618 L619 L620 L621 L622 A15 L623 L624 L625 L626 L627 L628 L629 L630 L631 L632 L633 L634 L635 L636 L637 L638 L639 L640 L641 L642 L643 L644 L645 L646 L647 L648 L649 L650 L651 L652 L653 L654 L655 L656 L657 L658 L659 L660 L661 L662 L663 L664 L665 L666 L667 L668 L669 L670 L671 L672 L673 L674 A16 L675 L676 L677 L678 L679 L680 L681 L682 L683 L684 L685 L686 L687 L688 L689 L690 L691 L692 L693 L694 L695 L696 L697 L698 L699 L700 L701 L702 L703 L704 L705 L706 L707 L708 L709 L710 L711 L712 L713 L714 L715 L716 L717 L718 L719 L720 L721 L722 L723 L724 L725 L726 A17 L727 L728 L729 L730 L731 L732 L733 L734 L735 L736 L737 L738 L739 L740 L741 L742 L743 L744 L745 L746 L747 L748 L749 L750 L751 L752 L753 L754 L755 L756 L757 L758 L759 L760 L761 L762 L763 L764 L765 L766 L767 L768 L769 L770 L771 L772 L773 L774 L775 L776 L777 L778 A18 L779
sketch "Sketch6" plane through (0, 0, 5.55) normal (0, 0, 1) x (1, 0, 0)
  circle A0 centre (37.5, 0) radius 2 construction
  line L0 (37.5, 0) -> (40.6, 0) construction
  line L1 (37.5, 0) -> (39.05, 2.6847) construction
  line L2 (37.5, 0) -> (35.95, 2.6847) construction
  line L3 (37.5, 0) -> (34.4, 0) construction
  line L4 (37.5, 0) -> (35.95, -2.6847) construction
  line L5 (37.5, 0) -> (39.05, -2.6847) construction
  line L6 (35.95, 2.6847) -> (39.05, 2.6847) construction
  line L7 (39.05, 2.6847) -> (40.6, 0) construction
  line L8 (40.6, 0) -> (39.05, -2.6847) construction
  line L9 (39.05, -2.6847) -> (35.95, -2.6847) construction
  line L10 (35.95, -2.6847) -> (34.4, 0) construction
  line L11 (34.4, 0) -> (35.95, 2.6847) construction
  line L12 (41.1774, 0) -> (39.3387, 3.1847)
  line L13 (39.3387, 3.1847) -> (35.6613, 3.1847)
  line L14 (35.6613, 3.1847) -> (33.8226, 0)
  line L15 (33.8226, 0) -> (35.6613, -3.1847)
  line L16 (35.6613, -3.1847) -> (39.3387, -3.1847)
  line L17 (39.3387, -3.1847) -> (41.1774, 0)
  point P0 (0, 0)
  dimension "d34" = 3.1
  dimension "d37" = 360
  dimension "d39" = 0.5
  constraints: 36 end point, 6 parallel, 2 coincident, 2 horizontal, 22 other
  measures "d34" distance of L0.start L0.end
  measures "d39" distance between parallel lines of L7 L12
extrude "Extrusion7" cut sketch "Sketch6" against normal blind 10
body "Solid1"
